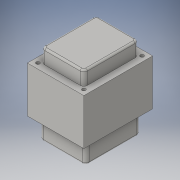
# Autodesk Inventor part: xmfr power
Saved by Autodesk Inventor 2016 (Build 200138000, 138)
## iProperties
Created: 2015-10-14
Part Number: xmfr power
Material: Generic
Document SubType Name: Modeling
Designer: jeremyhale
Density: 1 g/cm^3
Appearance: Default
Author: jeremyhale
Autodesk Inventor part; units mm, degrees
ref_plane "YZ Plane" through (0, 0, 0) normal (1, 0, 0) x (0, 1, 0)
ref_plane "XZ Plane" through (0, 0, 0) normal (0, 1, 0) x (-1, 0, 0)
ref_plane "XY Plane" through (0, 0, 0) normal (0, 0, 1) x (1, 0, 0)
sketch "Sketch1" plane through (0, 0, 0) normal (0, 1, 0) x (-1, 0, 0)
  line L0 (-50.8, 61.9125) -> (50.8, 61.9125)
  line L1 (50.8, 61.9125) -> (50.8, -61.9125)
  line L2 (50.8, -61.9125) -> (-50.8, -61.9125)
  line L3 (-50.8, -61.9125) -> (-50.8, 61.9125)
  line L4 (-50.8, 61.9125) -> (50.8, -61.9125) construction
  line L5 (50.8, 61.9125) -> (-50.8, -61.9125) construction
  point P0 (0, 0)
  dimension "d0" = 123.825
  dimension "d1" = 101.6
  constraints: 12 end point, 2 midpoint, 2 parallel, 1 horizontal, 1 perpendicular
  measures "d0" distance of L0.end L1.end
  measures "d1" distance of L1.end L2.end
extrude "Extrusion1" add sketch "Sketch1" along normal blind 82.55
sketch "Sketch2" plane through (0, 82.55, 0) normal (0, 1, 0) x (1, 0, 0)
  line L0 (31.75, -49.2125) -> (-31.75, -49.2125)
  line L1 (-38.1, -42.8625) -> (-38.1, 42.8625)
  line L2 (-31.75, 49.2125) -> (31.75, 49.2125)
  line L3 (38.1, 42.8625) -> (38.1, -42.8625)
  line L4 (38.1, -49.2125) -> (-38.1, 49.2125) construction
  line L5 (-38.1, -49.2125) -> (38.1, 49.2125) construction
  arc A0 (-38.1, -42.8625) -> (-31.75, -49.2125) centre (-31.75, -42.8625) ccw
  arc A1 (-31.75, 49.2125) -> (-38.1, 42.8625) centre (-31.75, 42.8625) ccw
  arc A2 (38.1, 42.8625) -> (31.75, 49.2125) centre (31.75, 42.8625) ccw
  arc A3 (31.75, -49.2125) -> (38.1, -42.8625) centre (31.75, -42.8625) ccw
  line L6 (-50.8, 61.9125) -> (-50.8, -61.9125) projected
  line L7 (50.8, 61.9125) -> (-50.8, 61.9125) projected
  point P0 (0, 0)
  dimension "d6" = 6.35
  dimension "d25" = 12.7
  dimension "d26" = 12.7
  constraints: 12 end point, 8 point on circle, 8 point on line, 8 tangent, 4 centre point, 3 equal radius, 2 midpoint, 2 parallel, 1 horizontal, 1 perpendicular
  measures "d6" radius of A0
  measures "d25" distance between parallel lines of L6 L1
  measures "d26" distance between parallel lines of L2 L7
extrude "Extrusion2" add sketch "Sketch2" along normal blind 25.4
fillet "Fillet1" radius 3.175 8 edges at (36.2401, 107.95, 47.3526) (38.1, 107.95, 0) (36.2401, 107.95, -47.3526) (0, 107.95, -49.2125) (-36.2401, 107.95, -47.3526) (-38.1, 107.95, 0) (-36.2401, 107.95, 47.3526) (0, 107.95, 49.2125)
hole "Hole1" at (41.275, 82.55, 52.3875) direction (0, -1, 0) diameter 6.35 end through all
pattern_linear "Rectangular Pattern1" count 2 spacing 104.775 along (0, 0, -1) count 2 spacing 82.55 along (-1, 0, 0) of "Hole1"
sketch "Sketch3" plane through (0, 0, 0) normal (0, -1, 0) x (1, 0, 0)
  line L0 (-34.925, -49.2125) -> (34.925, -49.2125)
  line L1 (41.275, -42.8625) -> (41.275, 42.8625)
  line L2 (34.925, 49.2125) -> (-34.925, 49.2125)
  line L3 (-41.275, 42.8625) -> (-41.275, -42.8625)
  line L4 (-41.275, -49.2125) -> (41.275, 49.2125) construction
  line L5 (41.275, -49.2125) -> (-41.275, 49.2125) construction
  line L6 (50.8, 61.9125) -> (-50.8, 61.9125) projected
  line L7 (50.8, -61.9125) -> (50.8, 61.9125) projected
  arc A0 (-34.925, 49.2125) -> (-41.275, 42.8625) centre (-34.925, 42.8625) ccw
  arc A1 (41.275, 42.8625) -> (34.925, 49.2125) centre (34.925, 42.8625) ccw
  arc A2 (34.925, -49.2125) -> (41.275, -42.8625) centre (34.925, -42.8625) ccw
  arc A3 (-41.275, -42.8625) -> (-34.925, -49.2125) centre (-34.925, -42.8625) ccw
  point P0 (0, 0)
  dimension "d27" = 12.7
  dimension "d28" = 9.525
  dimension "d29" = 6.35
  constraints: 12 end point, 8 point on circle, 8 point on line, 8 tangent, 4 centre point, 3 equal radius, 2 midpoint, 2 parallel, 1 horizontal, 1 perpendicular
  measures "d27" distance between parallel lines of L2 L6
  measures "d28" distance between parallel lines of L7 L1
  measures "d29" radius of A0
extrude "Extrusion3" add sketch "Sketch3" along normal blind 38.1
fillet "Fillet2" radius 3.175 8 edges at (-39.4151, -38.1, 47.3526) (-41.275, -38.1, 0) (-39.4151, -38.1, -47.3526) (0, -38.1, -49.2125) (39.4151, -38.1, -47.3526) (41.275, -38.1, 0) (39.4151, -38.1, 47.3526) (0, -38.1, 49.2125)
body "Solid1"
